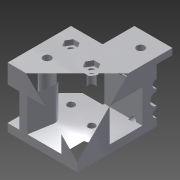
# Autodesk Inventor part: YAxisIdlerBlock
Saved by Autodesk Inventor 2015 (Build 190159000, 159)
## iProperties
Created: 2014-08-08
Part Number: YAxisIdlerBlock
Material: ABS Plastic
Document SubType Name: Modeling
Designer: Jack
Density: 1.06 g/cm^3
Appearance: Smooth - White
Author: Jack
Autodesk Inventor part; units mm, degrees
ref_plane "YZ Plane" through (0, 0, 0) normal (1, 0, 0) x (0, 1, 0)
ref_plane "XZ Plane" through (0, 0, 0) normal (0, 1, 0) x (-1, 0, 0)
ref_plane "XY Plane" through (0, 0, 0) normal (0, 0, 1) x (1, 0, 0)
sketch "Sketch1" plane through (0, 0, 0) normal (0, 0, 1) x (1, 0, 0)
  line L0 (0, 0) -> (44, 0)
  line L1 (44, 0) -> (44, 50)
  line L2 (44, 50) -> (20, 50)
  line L3 (20, 50) -> (20, 40)
  line L4 (20, 40) -> (0, 40)
  line L5 (0, 40) -> (0, 0)
  dimension "d0" = 44
  dimension "d1" = 50
  dimension "d2" = 24
  dimension "d3" = 10
  constraints: 12 end point, 4 perpendicular, 2 horizontal
  measures "d0" distance of L0.start L0.end
  measures "d1" distance of L0.end L1.end
  measures "d2" distance of L1.end L2.end
  measures "d3" distance of L2.end L3.end
extrude "Extrusion1" add sketch "Sketch1" along normal blind 5
sketch "Sketch2" plane through (0, 0, 5) normal (0, 0, 1) x (1, 0, 0)
  line L0 (44, 0) -> (44, 50) projected
  line L1 (44, 50) -> (20, 50) projected
  line L2 (20, 50) -> (20, 40) projected
  line L3 (20, 40) -> (44, 40)
  constraints: 2 end point, 1 perpendicular, 1 point on line
extrude "Extrusion2" add sketch "Sketch2" along normal blind 21
sketch "Sketch3" plane through (0, 0, 5) normal (0, 0, 1) x (1, 0, 0)
  line L0 (0, 40) -> (0, 0) projected
  line L1 (0, 0) -> (44, 0) projected
  circle A0 centre (10, 15) radius 5
  line L2 (7.5, 0) -> (5.072, 14.1547)
  line L3 (14.928, 14.1547) -> (12.5, 0)
  dimension "d8" = 10
  dimension "d9" = 15
  dimension "d10" = 10
  dimension "d11" = 7.5
  dimension "d12" = 5
  constraints: 4 end point, 2 point on circle, 2 point on line, 2 tangent, 1 centre point
  measures "d8" diameter of A0
  measures "d9" distance from line of L1 A0.centre
  measures "d10" distance from line of L0 A0.centre
  measures "d11" distance of L0.end L2.start
  measures "d12" distance of L2.start L3.end
extrude "Extrusion3" add sketch "Sketch3" along normal blind 21
sketch "Sketch4" plane through (0, 0, 5) normal (0, 0, 1) x (1, 0, 0)
  line L0 (12.5, 0) -> (44, 0) projected
  line L1 (44, 0) -> (44, 40) projected
  circle A0 centre (32, 25) radius 11
  line L2 (34, 14.1833) -> (34, 0)
  line L3 (42, 20.4174) -> (44, 20.4174)
  dimension "d15" = 22
  dimension "d16" = 25
  dimension "d17" = 12
  dimension "d18" = 10
  dimension "d23" = 2
  constraints: 4 end point, 2 perpendicular, 2 point on circle, 2 point on line, 1 centre point
  measures "d15" diameter of A0
  measures "d16" distance from line of L0 A0.centre
  measures "d17" distance from line of L1 A0.centre
  measures "d18" distance between parallel lines of L1 L2
  measures "d23" distance of L3.start L3.end
extrude "Extrusion4" add sketch "Sketch4" along normal blind 21 contours L2 A0 L3 L1 L0
sketch "Sketch5" plane through (0, 0, 26) normal (0, 0, 1) x (1, 0, 0)
  line L0 (44, 50) -> (20, 50) projected
  line L1 (20, 50) -> (20, 40) projected
  line L2 (20, 40) -> (44, 40) projected
  line L3 (44, 40) -> (44, 50) projected
  line L4 (42, 20.4174) -> (44, 20.4174) projected
  line L5 (44, 20.4174) -> (44, 40) projected
  line L6 (44, 40) -> (20, 40) projected
  line L7 (20, 40) -> (0, 40) projected
  line L8 (0, 40) -> (0, 0) projected
  line L9 (0, 0) -> (7.5, 0) projected
  line L10 (7.5, 0) -> (5.072, 14.1547) projected
  arc A0 (14.928, 14.1547) -> (5.072, 14.1547) centre (10, 15) ccw projected
  line L11 (14.928, 14.1547) -> (12.5, 0) projected
  line L12 (12.5, 0) -> (34, 0) projected
  line L13 (34, 0) -> (34, 14.1833) projected
  arc A1 (34, 14.1833) -> (42, 20.4174) centre (32, 25) ccw projected
  arc A2 (14.928, 14.1547) -> (5.072, 14.1547) centre (10, 15) ccw projected
  line L14 (5.072, 14.1547) -> (7.5, 0) projected
  line L15 (7.5, 0) -> (12.5, 0) projected
  line L16 (12.5, 0) -> (14.928, 14.1547) projected
  line L17 (44, 0) -> (44, 20.4174) projected
  line L18 (44, 20.4174) -> (42, 20.4174) projected
  arc A3 (34, 14.1833) -> (42, 20.4174) centre (32, 25) ccw projected
  line L19 (34, 14.1833) -> (34, 0) projected
  line L20 (34, 0) -> (44, 0) projected
extrude "Extrusion5" add sketch "Sketch5" along normal blind 12
sketch "Sketch6" plane through (0, 0, 38) normal (0, 0, 1) x (1, 0, 0)
  line L0 (20, 40) -> (0, 40) projected
  line L1 (0, 40) -> (0, 0) projected
  line L2 (0, 0) -> (44, 0) projected
  circle A0 centre (28, 25) radius 2.25
  circle A1 centre (10, 30) radius 2.25
  dimension "d24" = 4.5
  dimension "d26" = 25
  dimension "d28" = 10
  dimension "d29" = 10
  dimension "d60" = 28
  constraints: 2 centre point, 1 equal radius
  measures "d24" diameter of A0
  measures "d26" distance from line of L2 A0.centre
  measures "d28" distance from line of L0 A1.centre
  measures "d29" distance from line of L1 A1.centre
  measures "d60" distance from line of L1 A0.centre
extrude "Extrusion6" cut sketch "Sketch6" against normal up to surface (38 mm away)
sketch "Sketch7" plane through (0, 0, 0) normal (0, 0, -1) x (-1, 0, 0)
  circle A0 centre (-28, 25) radius 2.25 projected
  circle A1 centre (-10, 30) radius 2.25 projected
  circle A2 centre (-28, 25) radius 3.5
  circle A3 centre (-10, 30) radius 3.5
  dimension "d112" = 7
  dimension "d113" = 7
  constraints: 4 coincident, 2 centre point
  measures "d112" diameter of A2
  measures "d113" diameter of A3
extrude "Extrusion7" cut sketch "Sketch7" against normal blind 4
sketch "Sketch8" plane through (44, 0, 0) normal (1, 0, 0) x (0, 0, -1)
  line L0 (0, 50) -> (-38, 50)
  circle A0 centre (-15.5, 50) radius 4
  line L1 (-38, 0) -> (-38, 50) projected
  line L2 (0, 50) -> (-38, 50) projected
  dimension "d35" = 8
  dimension "d38" = 22.5
  constraints: 2 end point, 1 centre point, 1 point on line
  measures "d35" diameter of A0
  measures "d38" distance from line of L1 A0.centre
extrude "Extrusion8" cut sketch "Sketch8" against normal blind 20
sketch "Sketch9" plane through (0, 0, 38) normal (0, 0, 1) x (1, 0, 0)
  circle A0 centre (28, 25) radius 2.25 projected
  circle A1 centre (10, 30) radius 2.25 projected
  circle A2 centre (10, 30) radius 2.25 projected
  line L0 (14.0415, 30) -> (12.0207, 26.5)
  line L1 (12.0207, 26.5) -> (7.9793, 26.5)
  line L2 (7.9793, 26.5) -> (5.9585, 30)
  line L3 (5.9585, 30) -> (7.9793, 33.5)
  line L4 (7.9793, 33.5) -> (12.0207, 33.5)
  line L5 (12.0207, 33.5) -> (14.0415, 30)
  line L6 (32.0415, 25) -> (30.0207, 21.5)
  line L7 (30.0207, 21.5) -> (25.9793, 21.5)
  line L8 (25.9793, 21.5) -> (23.9585, 25)
  line L9 (23.9585, 25) -> (25.9793, 28.5)
  line L10 (25.9793, 28.5) -> (30.0207, 28.5)
  line L11 (30.0207, 28.5) -> (32.0415, 25)
  dimension "d110" = 7
  dimension "d111" = 7
  constraints: 24 end point, 2 coincident, 2 horizontal, 26 other
  measures "d110" distance between parallel lines of L1 L4
  measures "d111" distance between parallel lines of L7 L10
extrude "Extrusion9" cut sketch "Sketch9" against normal blind 3.2
sketch "Sketch10" plane through (0, 0, 0) normal (0, 0, -1) x (-1, 0, 0)
  arc A0 (-5.072, 14.1547) -> (-14.928, 14.1547) centre (-10, 15) ccw projected
  arc A1 (-5.072, 14.1547) -> (-14.928, 14.1547) centre (-10, 15) ccw projected
  circle A2 centre (-10, 15) radius 4.25
  dimension "d43" = 8.5
  constraints: 1 centre point, 1 coincident
  measures "d43" diameter of A2
extrude "Extrusion10" cut sketch "Sketch10" against normal blind 33
sketch "Sketch11" plane through (10, 15, 33) normal (0, 0, -1) x (-1, 0, 0)
  circle A0 centre (0, 0) radius 4.25 projected
  circle A1 centre (0, 0) radius 2.5
  point P0 (10, -15)
  dimension "d46" = 5
  constraints: 1 centre point, 1 coincident
  measures "d46" diameter of A1
extrude "Extrusion11" cut sketch "Sketch11" against normal up to next contours A1
sketch "Sketch12" plane through (20, 50, 0) normal (0, 1, 0) x (1, 0, 0)
  line L0 (24, 0) -> (24, -11.5) projected
  line L1 (24, -19.5) -> (4, -19.5) projected
  line L2 (0, 0) -> (0, -38) projected
  line L3 (24, -38) -> (0, -38) projected
  line L4 (24, -19.5) -> (24, -38) projected
  circle A0 centre (18, -5.5) radius 2
  circle A1 centre (18, -29.5) radius 2
  line L5 (4, -19.5) -> (4, -11.5) projected
  line L6 (4, -11.5) -> (24, -11.5) projected
  line L7 (24, 0) -> (24, -11.5) projected
  line L8 (24, 0) -> (0, 0) projected
  point P0 (-20, 0)
  dimension "d49" = 4
  dimension "d50" = 4
  dimension "d53" = 6
  dimension "d129" = 5.5
  dimension "d130" = 24
  constraints: 2 centre point, 1 vertical alignment
  measures "d49" diameter of A0
  measures "d50" diameter of A1
  measures "d53" distance from line of L0 A0.centre
  measures "d129" distance from line of L8 A0.centre
  measures "d130" distance of A1.centre A0.centre
extrude "Extrusion12" cut sketch "Sketch12" against normal up to surface (10 mm away) contours A0 | A1
sketch "Sketch15" plane through (20, 50, 0) normal (0, 1, 0) x (1, 0, 0)
  line L0 (24, 0) -> (0, 0) projected
  line L1 (0, 0) -> (0, -38) projected
  line L2 (24, -38) -> (0, -38) projected
  line L3 (4, 0) -> (4, -38)
  point P0 (4, -19.5)
  point P1 (-20, 0)
  constraints: 3 point on line, 2 end point, 1 perpendicular
extrude "Extrusion15" add sketch "Sketch15" along normal blind 10
sketch "Sketch16" plane through (24, 0, 0) normal (1, 0, 0) x (0, 0, -1)
  line L0 (-38, 60) -> (0, 60) projected
  line L1 (-38, 50) -> (-38, 60) projected
  line L2 (-19.5, 50) -> (-38, 50) projected
  line L3 (-34, 60) -> (-34, 50)
  point P0 (0, 0)
  dimension "d72" = 4
  constraints: 2 end point, 2 point on line, 1 vertical
  measures "d72" distance between parallel lines of L1 L3
extrude "Extrusion16" add sketch "Sketch16" along normal up to surface (20 mm away)
sketch "Sketch17" plane through (24, 0, 0) normal (1, 0, 0) x (0, 0, -1)
  arc A0 (-19.5, 50) -> (-11.5, 50) centre (-15.5, 50) ccw projected
  line L0 (-34, 60) -> (0, 60) projected
  circle A1 centre (-23.5, 50) radius 2.5
  circle A2 centre (-7.5, 50) radius 2.5
  point P0 (0, 0)
  dimension "d75" = 5
  dimension "d76" = 5
  dimension "d77" = 10
  dimension "d78" = 8
  dimension "d79" = 8
  constraints: 2 centre point, 1 horizontal alignment
  measures "d75" diameter of A1
  measures "d76" diameter of A2
  measures "d77" distance from line of L0 A2.centre
  measures "d78" distance of A0.centre A1.centre
  measures "d79" distance of A0.centre A2.centre
extrude "Extrusion17" cut sketch "Sketch17" against normal up to next
sketch "Sketch18" plane through (24, 0, 0) normal (-1, 0, 0) x (0, 0, 1)
  arc A0 (21, 50) -> (26, 50) centre (23.5, 50) ccw projected
  line L0 (5, 50) -> (10, 50) projected
  arc A1 (5, 50) -> (10, 50) centre (7.5, 50) ccw projected
  circle A2 centre (7.5, 50) radius 4.25
  circle A3 centre (23.5, 50) radius 4.25
  point P0 (0, 0)
  point P1 (34, 52.4495)
  dimension "d82" = 8.5
  dimension "d83" = 8.5
  constraints: 2 centre point, 2 coincident, 1 other
  measures "d82" diameter of A2
  measures "d83" diameter of A3
extrude "Extrusion18" cut sketch "Sketch18" against normal blind 9 contours L0 A1 | A2 | A3
sketch "Sketch19" plane through (44, 0, 0) normal (1, 0, 0) x (0, 0, -1)
  circle A0 centre (-23.5, 50) radius 2.5 projected
  circle A1 centre (-23.5, 50) radius 2.5 projected
  circle A2 centre (-7.5, 50) radius 2.5 projected
  circle A3 centre (-7.5, 50) radius 2.5 projected
extrude "Extrusion19" cut sketch "Sketch19" against normal blind 13
sketch "Sketch20" plane through (24, 50, 34) normal (0, 0, -1) x (-1, 0, 0)
  line L0 (0, 10) -> (-20, 10) projected
  circle A0 centre (-10, 0) radius 2.5
  line L1 (0, 10) -> (0, 0) projected
  point P0 (24, -50)
  point P1 (0, 2.4109)
  dimension "d88" = 5
  dimension "d89" = 10
  dimension "d109" = 10
  constraints: 1 centre point
  measures "d88" diameter of A0
  measures "d89" distance from line of L0 A0.centre
  measures "d109" distance from line of L1 A0.centre
extrude "Extrusion20" cut sketch "Sketch20" against normal up to next
sketch "Sketch23" plane through (24, 50, 34) normal (0, 0, -1) x (-1, 0, 0)
  arc A0 (-7.5, 0) -> (-12.5, 0) centre (-10, 0) ccw projected
  circle A1 centre (-10, 0) radius 1.8
  point P0 (24, -50)
  point P1 (-9, 2.2913)
  point P2 (-9.5, 2.4495)
  point P3 (-10.5, 2.4495)
  dimension "d98" = 3.6
  constraints: 1 centre point, 1 coincident
  measures "d98" diameter of A1
extrude "Extrusion23" cut sketch "Sketch23" along normal up to surface (34 mm away)
sketch "Sketch28" plane through (20, 40, 5) normal (0, -1, 0) x (1, 0, 0)
  circle A0 centre (18, 0.5) radius 2 projected
  line L0 (24, 0) -> (0, 0) projected
  line L1 (24, 0) -> (24, 21) projected
  line L2 (0, 21) -> (24, 21) projected
  line L3 (0, 0) -> (0, 21) projected
  point P0 (-20, -5)
extrude "Extrusion26" cut sketch "Sketch28" against normal blind 1 contours A0 L0 L3 L2 L1
body "Solid1"
